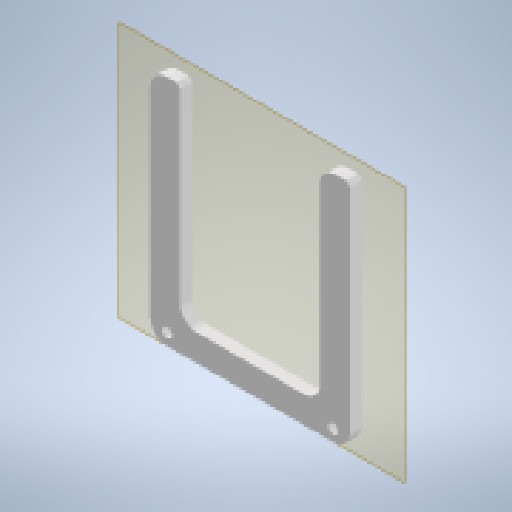
# Autodesk Inventor part: соединялка
Saved by Autodesk Inventor 2024.2 (Build 282272000, 272)
## iProperties
Created: 2026-01-07
Part Number: соединялка
Material: Типовые
Document SubType Name: Modeling
Designer: Service
Density: 1 g/cm^3
Appearance: По умолчанию
Author: Service
Autodesk Inventor part; units mm, degrees
ref_plane "YZ Plane" through (0, 0, 0) normal (1, 0, 0) x (0, 1, 0)
ref_plane "XZ Plane" through (0, 0, 0) normal (0, 1, 0) x (-1, 0, 0)
ref_plane "XY Plane" through (0, 0, 0) normal (0, 0, 1) x (1, 0, 0)
ref_plane "РабПлоскость1" through (0, 0, 0) normal (0, 0, 1) x (1, 0, 0)
sketch "Эскиз1" plane through (0, 0, 0) normal (0, 0, 1) x (1, 0, 0)
  line L0 (-54.6061, 570.3445) -> (-45.6061, 570.3445) projected
  line L1 (-45.6061, 570.3445) -> (-45.6061, 587.3445) projected
  line L2 (-45.6061, 587.3445) -> (-54.6061, 587.3445) projected
  line L3 (-54.6061, 587.3445) -> (-54.6061, 627.3645) projected
  line L4 (-54.6061, 627.3645) -> (-114.6061, 627.3645) projected
  line L5 (-114.6061, 627.3645) -> (-114.6061, 587.3445) projected
  line L6 (-114.6061, 587.3445) -> (-123.6061, 587.3445) projected
  line L7 (-123.6061, 587.3445) -> (-123.6061, 570.3445) projected
  line L8 (-123.6061, 570.3445) -> (-114.6061, 570.3445) projected
  line L9 (-114.6061, 570.3445) -> (-114.6061, 557.3645) projected
  line L10 (-114.6061, 557.3645) -> (-54.6061, 557.3645) projected
  line L11 (-54.6061, 557.3645) -> (-54.6061, 570.3445) projected
  line L12 (-48.6061, 575.3445) -> (-51.6061, 575.3445) projected
  line L13 (-51.6061, 575.3445) -> (-51.6061, 582.3445) projected
  line L14 (-51.6061, 582.3445) -> (-48.6061, 582.3445) projected
  line L15 (-48.6061, 582.3445) -> (-48.6061, 575.3445) projected
  line L16 (-117.6061, 582.3445) -> (-117.6061, 575.3445) projected
  line L17 (-117.6061, 575.3445) -> (-120.6061, 575.3445) projected
  line L18 (-120.6061, 575.3445) -> (-120.6061, 582.3445) projected
  line L19 (-120.6061, 582.3445) -> (-117.6061, 582.3445) projected
  circle A0 centre (-97.1061, 577.3245) radius 2.575 projected
  circle A1 centre (-72.1061, 577.3245) radius 2.575 projected
  circle A2 centre (-72.1061, 617.3645) radius 2.575 projected
  circle A3 centre (-97.1061, 617.3645) radius 2.575 projected
  circle A4 centre (-109.6061, 560.8645) radius 1.5 projected
  circle A5 centre (-59.6061, 560.8645) radius 1.5 projected
  circle A6 centre (-106.1061, 572.3645) radius 1 projected
  circle A7 centre (-63.1061, 572.3645) radius 1 projected
  circle A8 centre (-106.1061, 587.3645) radius 1 projected
  circle A9 centre (-63.1061, 587.3645) radius 1 projected
  circle A10 centre (-106.1061, 602.3645) radius 1 projected
  circle A11 centre (-63.1061, 602.3645) radius 1 projected
  circle A12 centre (-106.1061, 617.3645) radius 1 projected
  circle A13 centre (-63.1061, 617.3645) radius 1 projected
  line L20 (-59.6061, 627.3645) -> (-54.6061, 627.3645)
  line L21 (-54.6061, 627.3645) -> (-54.6061, 557.3645)
  line L22 (-54.6061, 557.3645) -> (-59.6061, 557.3645)
  line L23 (-59.6061, 557.3645) -> (-59.6061, 627.3645)
  line L24 (-54.6061, 557.3645) -> (-114.6061, 557.3645)
  line L25 (-114.6061, 557.3645) -> (-114.6061, 565.3645)
  line L26 (-114.6061, 565.3645) -> (-54.6061, 565.3645)
  line L27 (-54.6061, 565.3645) -> (-54.6061, 557.3645)
  line L28 (-114.6061, 557.3645) -> (-109.6061, 557.3645)
  line L29 (-109.6061, 557.3645) -> (-109.6061, 627.3645)
  line L30 (-109.6061, 627.3645) -> (-114.6061, 627.3645)
  line L31 (-114.6061, 627.3645) -> (-114.6061, 557.3645)
  circle A14 centre (-59.6061, 560.8645) radius 1.5
  circle A15 centre (-109.6061, 560.8645) radius 1.5
  point P0 (0, 0)
  point P1 (-59.6061, 565.3645)
  point P2 (-109.6061, 565.3645)
  dimension "d0" = 5
  dimension "d1" = 5
  dimension "d2" = 8
  constraints: 24 end point, 6 parallel, 3 horizontal, 3 perpendicular, 3 point on line, 2 centre point, 2 coincident, 2 concentric
  measures "d0" distance between parallel lines of L5 L29
  measures "d1" distance between parallel lines of L21 L23
  measures "d2" distance between parallel lines of L10 L26
extrude "Выдавливание1" add sketch "Эскиз1" along normal blind 3.65 contours L11 L26 L23 L4 L3 L21 | L11 L10 L23 A5 L26 | L23 A5 L10 L29 A4 L26 | L29 A4 L10 L9 L26 | L26 L9 L31 L5 L4 L29
fillet "Сопряжение грани1" radius 5 1 edges at (-109.6061, 565.3645, 1.825)
fillet "Сопряжение грани2" radius 5 1 edges at (-59.6061, 565.3645, 1.825)
fillet "Сопряжение грани3" radius 5 1 edges at (-59.6061, 627.3645, 1.825)
fillet "Сопряжение грани4" radius 5 1 edges at (-114.6061, 627.3645, 1.825)
feature "Сопряжение грани5" [suppressed]
feature "Сопряжение грани6" [suppressed]
fillet "Сопряжение грани7" radius 5 1 edges at (-54.6061, 557.3645, 1.825)
fillet "Сопряжение грани8" radius 5 1 edges at (-114.6061, 557.3645, 1.825)
